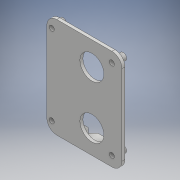
# Autodesk Inventor part: Base
Saved by Autodesk Inventor 2019 (Build 230136000, 136)
## iProperties
Created: 2016-12-12
Part Number: Base
Material: Genérico
Document SubType Name: Modeling
Designer: Mario
Density: 1 g/cm^3
Appearance: Por defecto
Author: Mario
Autodesk Inventor part; units mm, degrees
sketch "Sketch1" plane through (0, 0, 0) normal (0, 1, 0) x (-1, 0, 0)
  line L0 (45, 40) -> (45, -40)
  circle A0 centre (0, 26.37) radius 12
  circle A1 centre (0, -26.38) radius 12
  line L1 (45, 40) -> (45, 40)
  line L2 (45, -40) -> (45, -40)
  line L3 (45, 40) -> (45, 40)
  line L4 (45, -40) -> (45, -40)
  line L5 (35, -50) -> (-20, -50)
  line L6 (-30, -40) -> (-30, 40)
  line L7 (-20, 50) -> (35, 50)
  arc A2 (45, 40) -> (35, 50) centre (35, 40) ccw
  arc A3 (-20, 50) -> (-30, 40) centre (-20, 40) ccw
  arc A4 (-30, -40) -> (-20, -50) centre (-20, -40) ccw
  arc A5 (35, -50) -> (45, -40) centre (35, -40) ccw
  point P0 (0, 0)
  dimension "d4" = 24
  dimension "d5" = 24
  constraints: 16 end point, 8 point on circle, 8 tangent, 6 centre point, 3 equal radius, 3 vertical, 2 perpendicular, 1 horizontal
  measures "d4" diameter of A0
  measures "d5" diameter of A1
extrude "Extrusion1" add sketch "Sketch1" along normal blind 3
sketch "Sketch4" plane through (0, 3, 0) normal (0, 1, 0) x (1, 0, 0)
  arc A0 (11.7028, -23.716) -> (10.7681, -21.0741) centre (14, -21.417) ccw
  arc A1 (10.7681, -31.6659) -> (11.7028, -29.024) centre (14, -31.323) ccw
  circle A2 centre (0, -26.37) radius 12
  circle A3 centre (-34.15, -21.417) radius 3.25
  circle A4 centre (-34.15, -31.323) radius 3.25
  circle A5 centre (0, 26.38) radius 12
  arc A6 (11.7028, 29.034) -> (10.7681, 31.6759) centre (14, 31.333) ccw
  arc A7 (10.7681, 21.0841) -> (11.7028, 23.726) centre (14, 21.427) ccw
  circle A8 centre (-34.15, 31.333) radius 3.25
  circle A9 centre (-34.15, 21.427) radius 3.25
  arc A10 (11.7028, 29.034) -> (10.7681, 31.6759) centre (14, 31.333) ccw
  arc A11 (10.7681, 21.0841) -> (11.7028, 23.726) centre (14, 21.427) ccw
  circle A12 centre (14, -31.323) radius 2.1
  circle A13 centre (14, -21.417) radius 2.1
  circle A14 centre (-34.15, -21.417) radius 2.1
  circle A15 centre (-34.15, -31.323) radius 2.1
  circle A16 centre (14, 21.427) radius 2.1
  circle A17 centre (14, 31.333) radius 2.1
  circle A18 centre (-34.15, 31.333) radius 2.1
  circle A19 centre (-34.15, 21.427) radius 2.1
  point P0 (0, 0)
  dimension "d8" = 6.5
  dimension "d9" = 6.5
  dimension "d10" = 6.5
  dimension "d11" = 6.5
  dimension "d14" = 6.5
  dimension "d15" = 6.5
  dimension "d16" = 6.5
  dimension "d17" = 6.5
  dimension "d85" = 4.2
  dimension "d86" = 4.2
  dimension "d87" = 4.2
  dimension "d88" = 4.2
  dimension "d89" = 4.2
  dimension "d90" = 4.2
  dimension "d91" = 4.2
  dimension "d92" = 4.2
  constraints: 20 centre point, 20 point on circle, 3 coincident
  measures "d8" diameter of A0
  measures "d9" diameter of A1
  measures "d10" diameter of A3
  measures "d11" diameter of A4
  measures "d14" diameter of A6
  measures "d15" diameter of A7
  measures "d16" diameter of A8
  measures "d17" diameter of A9
  measures "d85" diameter of A12
  measures "d86" diameter of A13
  measures "d87" diameter of A14
  measures "d88" diameter of A15
  measures "d89" diameter of A16
  measures "d90" diameter of A17
  measures "d91" diameter of A18
  measures "d92" diameter of A19
sketch "Sketch12" plane through (0, 3, 0) normal (0, 1, 0) x (1, 0, 0)
  arc A0 (-45, -40) -> (-40, -50) centre (-40, -40) ccw projected
  arc A1 (-40, 50) -> (-45, 40) centre (-40, 40) ccw projected
  arc A2 (40, -50) -> (50, -40) centre (40, -40) ccw projected
  arc A3 (50, 40) -> (40, 50) centre (40, 40) ccw projected
  circle A4 centre (-40, -40) radius 3.5
  circle A5 centre (-40, 40) radius 3.5
  circle A6 centre (20, 40) radius 3.5
  circle A7 centre (20, -40) radius 3.5
  point P0 (0, 0)
  dimension "d66" = 7
  dimension "d67" = 7
  dimension "d68" = 7
  dimension "d69" = 7
  constraints: 4 centre point, 1 coincident, 2 other
  measures "d66" diameter of A4
  measures "d67" diameter of A5
  measures "d68" diameter of A6
  measures "d69" diameter of A7
extrude "Extrusion10" add sketch "Sketch12" along normal blind 40.2
sketch "Sketch13" plane through (0, 0, 0) normal (0, -1, 0) x (1, 0, 0)
  circle A0 centre (-40, 40) radius 3.5 projected
  circle A1 centre (-40, -40) radius 3.5 projected
  circle A2 centre (20, -40) radius 3.5 projected
  circle A3 centre (20, 40) radius 3.5 projected
  circle A4 centre (-40, 40) radius 2.5
  circle A5 centre (20, 40) radius 2.5
  circle A6 centre (20, -40) radius 2.5
  circle A7 centre (-40, -40) radius 2.5
  point P0 (0, 0)
  dimension "d72" = 5
  dimension "d73" = 5
  dimension "d74" = 5
  dimension "d75" = 5
  constraints: 4 centre point, 1 coincident
  measures "d72" diameter of A4
  measures "d73" diameter of A5
  measures "d74" diameter of A6
  measures "d75" diameter of A7
extrude "Extrusion11" cut sketch "Sketch13" against normal blind 40.2 contours A4 | A5 | A6 | A7
sketch "Sketch15" plane through (0, 0, 0) normal (0, -1, 0) x (1, 0, 0)
  circle A0 centre (20, -40) radius 2.5 projected
  circle A1 centre (20, -40) radius 1.5
  circle A2 centre (-40, -40) radius 2.5 projected
  circle A3 centre (-40, 40) radius 2.5 projected
  circle A4 centre (20, 40) radius 2.5 projected
  circle A5 centre (-40, -40) radius 1.5
  circle A6 centre (40, 40) radius 1.5
  circle A7 centre (-40, 40) radius 1.5
  point P0 (0, 0)
  dimension "d78" = 3
  dimension "d79" = 3
  dimension "d80" = 3
  dimension "d81" = 3
  constraints: 4 centre point, 1 coincident
  measures "d78" diameter of A1
  measures "d79" diameter of A5
  measures "d80" diameter of A6
  measures "d81" diameter of A7
extrude "Extrusion12" cut sketch "Sketch15" against normal blind 45 contours A1 | A5 | A6 | A7
extrude "Extrusion13" add sketch "Sketch4" along normal blind 18.75 contours A2 A0 | A2 A1 | A3 | A4 | A5 A6 | A7 A5 | A8 | A9
sketch "Sketch16" plane through (0, 3, 0) normal (0, 1, 0) x (1, 0, 0)
  arc A0 (10.7681, -31.6659) -> (11.7028, -29.024) centre (14, -31.323) ccw projected
  line L0 (13.1326, -28.8149) -> (14.8075, -28.8149)
  line L1 (14.8075, -28.8149) -> (14.8075, -23.8271)
  line L2 (14.8075, -23.8271) -> (13.1326, -23.8271)
  line L3 (13.1326, -23.8271) -> (13.1326, -28.8149)
  circle A1 centre (-34.15, -31.323) radius 2.1 projected
  circle A2 centre (-34.15, 21.427) radius 2.1 projected
  circle A3 centre (14, 21.427) radius 2.1 projected
  line L4 (-35.0173, -28.8149) -> (-33.3425, -28.8149)
  line L5 (-33.3425, -28.8149) -> (-33.3425, -23.8271)
  line L6 (-33.3425, -23.8271) -> (-35.0173, -23.8271)
  line L7 (-35.0173, -23.8271) -> (-35.0173, -28.8149)
  line L8 (-35.0173, 23.9351) -> (-33.3425, 23.9351)
  line L9 (-33.3425, 23.9351) -> (-33.3425, 28.9229)
  line L10 (-33.3425, 28.9229) -> (-35.0173, 28.9229)
  line L11 (-35.0173, 28.9229) -> (-35.0173, 23.9351)
  line L12 (13.1326, 23.9351) -> (14.8075, 23.9351)
  line L13 (14.8075, 23.9351) -> (14.8075, 28.9229)
  line L14 (14.8075, 28.9229) -> (13.1326, 28.9229)
  line L15 (13.1326, 28.9229) -> (13.1326, 23.9351)
  point P0 (0, 0)
  constraints: 32 end point, 8 parallel, 4 horizontal, 4 perpendicular
extrude "Extrusion14" add sketch "Sketch16" along normal blind 15 contours L1 L0 L3 A0 | A0 L3 L2 L1 | L7 L6 L5 L4 | L11 L10 L9 L8 | L15 L14 L13 L12
ref_plane "Work Plane1" through (25.7052, 3, 40.0426) normal (0, 0, 1) x (1, 0, 0)
sketch "Sketch17" plane through (25.7052, 3, 40.0426) normal (0, 0, 1) x (1, 0, 0)
  line L0 (-9.2052, 0) -> (-2.2052, 0) projected
  line L1 (-9.2052, 0) -> (-8.2052, 0)
  line L2 (-8.2052, 0) -> (-8.2052, 30)
  line L3 (-8.2052, -3) -> (-8.2052, 37.2) projected
  line L4 (-8.2052, 0) -> (-38.2052, 0)
  line L5 (-38.2052, 0) -> (-8.2052, 30)
  line L6 (-69.2052, 0) -> (-62.2052, 0) projected
  line L7 (-62.2052, 0) -> (-63.2052, 0)
  line L8 (-63.2052, 0) -> (-63.2052, 30)
  line L9 (-63.2052, -3) -> (-63.2052, 37.2) projected
  line L10 (-62.2052, 0) -> (-32.2052, 0)
  line L11 (-32.2052, 0) -> (-63.2052, 30)
  point P0 (-25.7052, -3)
  dimension "d100" = 1
  dimension "d101" = 30
  dimension "d102" = 30
  dimension "d103" = 1
  dimension "d104" = 30
  dimension "d105" = 30
  constraints: 16 end point, 4 point on line, 1 horizontal, 1 perpendicular
  measures "d100" distance of L0.start L1.end
  measures "d101" distance of L1.end L2.end
  measures "d102" distance of L1.end L4.end
  measures "d103" distance of L6.end L7.end
  measures "d104" distance of L7.end L8.end
  measures "d105" distance of L6.end L10.end
extrude "Extrusion15" add sketch "Sketch17" along normal blind 1 and the other way blind 1
ref_plane "Work Plane2" through (-22.2948, 3, -39.9574) normal (0, 0, -1) x (-1, 0, 0)
sketch "Sketch18" plane through (-22.2948, 3, -39.9574) normal (0, 0, -1) x (-1, 0, 0)
  line L0 (14.2052, 0) -> (21.2052, 0) projected
  line L1 (14.2052, 0) -> (15.2052, 0)
  line L2 (15.2052, 0) -> (15.2052, 30)
  line L3 (14.2052, 0) -> (-15.7948, 0)
  line L4 (14.2052, 0) -> (14.2052, 40.2) projected
  line L5 (14.2052, 0) -> (44.2052, 0) construction
  line L6 (-15.7948, 0) -> (15.2052, 30)
  line L7 (-45.7948, 0) -> (-38.7948, 0) projected
  line L8 (-38.7948, 0) -> (-39.7948, 0)
  line L9 (-39.7948, -3) -> (-39.7948, 37.2) projected
  line L10 (-39.7948, 0) -> (-39.7948, 30)
  line L11 (-38.7948, 0) -> (-8.7948, 0)
  line L12 (-8.7948, 0) -> (-39.7948, 30)
  point P0 (-22.2948, -3)
  dimension "d111" = 1
  dimension "d112" = 30
  dimension "d114" = 30
  dimension "d116" = 1
  dimension "d117" = 30
  dimension "d118" = 90
  dimension "d119" = 30
  constraints: 18 end point, 3 perpendicular, 2 collinear, 2 point on line, 1 horizontal
  measures "d111" distance of L0.start L1.end
  measures "d112" distance of L1.end L2.end
  measures "d114" distance of L0.start L3.end
  measures "d116" distance of L7.end L8.end
  measures "d117" distance of L8.end L10.end
  measures "d118" angle of L8 L10
  measures "d119" distance of L7.end L11.end
extrude "Extrusion16" add sketch "Sketch18" along normal blind 1 and the other way blind 1
ref_plane "Plano de trabajo3" through (-35.2948, 3, 12.2426) normal (1, 0, 0) x (0, 0, -1)
sketch "Sketch19" plane through (-35.2948, 3, 12.2426) normal (1, 0, 0) x (0, 0, -1)
  line L0 (24, 0) -> (0, 0)
  line L1 (24, 0) -> (24, 1.79)
  line L2 (0, 0) -> (0, 1.79)
  line L3 (24, 0) -> (0, 0)
  line L4 (0, 0) -> (0, 1.79)
  line L5 (0, 0) -> (0, 1.79)
  line L6 (0, 1.79) -> (24, 1.79)
  line L7 (24, 0) -> (24, 1.79)
  line L8 (24, 0) -> (0, 0)
  point P0 (12.2426, -3)
  dimension "d124" = 1.79
  constraints: 18 end point
  measures "d124" distance of L2.end L0.end
extrude "Extrusion17" add sketch "Sketch19" along normal blind 60
sketch "Boceto20" plane through (0, 0, 0) normal (0, -1, 0) x (1, 0, 0)
  circle A0 centre (20, 40) radius 1.5
  dimension "d134" = 3
  constraints: 1 centre point, 1 coincident
  measures "d134" diameter of A0
extrude "Extrusión18" cut sketch "Boceto20" against normal blind 50
sketch "Boceto21" plane through (-34.15, 21.75, 21.417) normal (0, 1, 0) x (1, 0, 0)
  line L0 (-4.6077, 4.0688) -> (55.0118, 4.0688)
  line L1 (55.0118, 4.0688) -> (55.0118, -14.3175)
  line L2 (55.0118, -14.3175) -> (-4.6077, -14.3175)
  line L3 (-4.6077, -14.3175) -> (-4.6077, 4.0688)
  line L4 (-4.6077, 36.816) -> (54.2502, 36.816)
  line L5 (54.2502, 36.816) -> (54.2502, 56.8342)
  line L6 (54.2502, 56.8342) -> (-4.6077, 56.8342)
  line L7 (-4.6077, 56.8342) -> (-4.6077, 36.816)
  point P0 (34.15, 21.417)
  constraints: 16 end point, 4 parallel, 2 horizontal, 2 perpendicular, 1 point on line
extrude "Extrusión19" cut sketch "Boceto21" against normal blind 11.75
sketch "Boceto22" plane through (-40, 43.2, 40) normal (0, 1, 0) x (1, 0, 0)
  line L0 (-10.3612, -16.6308) -> (76.4591, -16.6308)
  line L1 (76.4591, -16.6308) -> (76.4591, 125.6618)
  line L2 (76.4591, 125.6618) -> (-10.3612, 125.6618)
  line L3 (-10.3612, 125.6618) -> (-10.3612, -16.6308)
  point P0 (40, 40)
  constraints: 8 end point, 2 parallel, 1 horizontal, 1 perpendicular
extrude "Extrusión20" cut sketch "Boceto22" against normal blind 32
body "Solid1"
